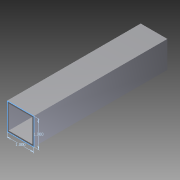
# Autodesk Inventor part: latch mount point
Saved by Autodesk Inventor 2011 SP1 (Build 150282100, 282)
## iProperties
Created: 2013-01-14
Part Number: latch mount point
Document SubType Name: Modeling
Designer: 355283
Density: 1 g/cm^3
Author: 355283
Autodesk Inventor part; units mm, degrees
ref_plane "YZ Plane" through (0, 0, 0) normal (1, 0, 0) x (0, 1, 0)
ref_plane "XZ Plane" through (0, 0, 0) normal (0, 1, 0) x (-1, 0, 0)
sketch "Sketch1" plane through (0, 0, 0) normal (0, 0, 1) x (1, 0, 0)
  line L0 (0, 0) -> (25.4, 0)
  line L1 (25.4, 0) -> (25.4, -25.4)
  line L2 (25.4, -25.4) -> (0, -25.4)
  line L3 (0, -25.4) -> (0, 0)
  dimension "d0" = 25.4
  dimension "d1" = 25.4
  constraints: 8 end point, 2 parallel, 1 horizontal, 1 perpendicular
  measures "d0" distance of L1.end L2.end
  measures "d1" distance of L0.end L1.end
ref_plane "Work Plane1" through (0, 0, 0) normal (0, 0, -1) x (1, 0, 0)
sketch "Sketch2" plane through (0, 0, 0) normal (0, 0, -1) x (1, 0, 0)
  line L0 (1.524, 1.524) -> (23.876, 1.524)
  line L1 (23.876, 1.524) -> (23.876, 23.876)
  line L2 (23.876, 23.876) -> (1.524, 23.876)
  line L3 (1.524, 23.876) -> (1.524, 1.524)
  line L4 (0, 25.4) -> (0, 0) projected
  line L5 (0, 0) -> (25.4, 0) projected
  line L6 (25.4, 25.4) -> (0, 25.4) projected
  line L7 (25.4, 0) -> (25.4, 25.4) projected
  dimension "margin" = 1.524
  dimension "d3" = 1.524
  dimension "d4" = 1.524
  dimension "d5" = 1.524
  constraints: 8 end point, 2 parallel, 1 horizontal, 1 perpendicular
  measures "margin" distance between parallel lines of L4 L3
  measures "d3" distance between parallel lines of L7 L1
  measures "d4" distance between parallel lines of L5 L0
  measures "d5" distance between parallel lines of L6 L2
extrude "Extrusion1" add sketch "Sketch2" along normal blind 127
equation "\"d3\" = margin"
equation "\"d4\" = margin"
equation "\"d5\" = margin"
body "Solid1"
